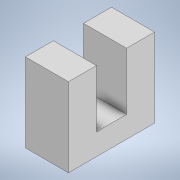
# Autodesk Inventor part: Encoder
Saved by Autodesk Inventor 2021 (Build 250183000, 183)
## iProperties
Created: 2022-12-02
Part Number: Encoder
Material: Genérico
Document SubType Name: Modeling
Designer: sergi
Density: 1 g/cm^3
Appearance: Valor por defecto
Author: sergi
Autodesk Inventor part; units mm, degrees
ref_plane "YZ Plane" through (0, 0, 0) normal (1, 0, 0) x (0, 1, 0)
ref_plane "XZ Plane" through (0, 0, 0) normal (0, 1, 0) x (-1, 0, 0)
ref_plane "XY Plane" through (0, 0, 0) normal (0, 0, 1) x (1, 0, 0)
sketch "Boceto1" plane through (0, 0, 0) normal (1, 0, 0) x (0, 1, 0)
  line L0 (0, 0) -> (0, -2.05)
  line L1 (0, -2.05) -> (8, -2.05)
  line L2 (8, -2.05) -> (8, -5.95)
  line L3 (8, -5.95) -> (-3, -5.95)
  line L4 (-3, -5.95) -> (-3, 6.05)
  line L5 (-3, 6.05) -> (8, 6.05)
  line L6 (8, 6.05) -> (8, 2.15)
  line L7 (8, 2.15) -> (0, 2.15)
  line L8 (0, 2.15) -> (0, 0)
  dimension "d0" = 2.05
  dimension "d1" = 8
  dimension "d2" = 3.9
  dimension "d3" = 11
  dimension "d4" = 12
  dimension "d5" = 11
  dimension "d6" = 3.9
  constraints: 18 end point, 5 perpendicular, 3 point on line, 1 collinear, 1 vertical
  measures "d0" distance of L0.start L0.end
  measures "d1" distance of L0.end L1.end
  measures "d2" distance of L1.end L2.end
  measures "d3" distance of L2.end L3.end
  measures "d4" distance of L3.end L4.end
  measures "d5" distance of L4.end L5.end
  measures "d6" distance of L5.end L6.end
extrude "Extrusión1" add sketch "Boceto1" along normal blind 6
